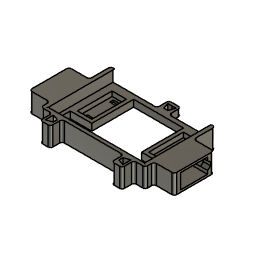
RobotV3 (Autodesk Fusion 360 design; units mm, degrees)
Autodesk Fusion 360 part; units mm, degrees
note: some values were not read from the file. Set by a fixed rule: which sketch regions a step uses.
sketch "Sketch1" plane through (0, 0, 0) normal (0, 0, 1) x (1, 0, 0)
  line L0 (0, 0) -> (83.7, 0)
  line L1 (83.7, 0) -> (83.7, 54.9)
  line L2 (83.7, 54.9) -> (0, 54.9)
  line L3 (0, 54.9) -> (0, 0)
  line L4 (0, 27.45) -> (0, 33.45)
  line L5 (0, 33.45) -> (-1.8, 33.45)
  line L6 (-1.8, 33.45) -> (-25.3, 33.45)
  line L7 (-25.3, 33.45) -> (-25.3, 10.78)
  line L8 (-25.3, 10.78) -> (0, 10.78)
  line L9 (-1.8, 33.45) -> (-1.8, 10.78)
  line L10 (-25.3, 33.45) -> (-25.3, 38.65)
  line L11 (-25.3, 38.65) -> (0, 38.65)
  line L12 (-1.8, 33.45) -> (-1.8, 38.65)
  line L13 (-25.3, 38.65) -> (0, 38.65)
  line L14 (0, 38.65) -> (0, 40.45)
  line L15 (0, 40.45) -> (-25.3, 40.45)
  line L16 (-25.3, 40.45) -> (-25.3, 38.65)
  line L17 (-21.6, 33.45) -> (-18.8, 33.45)
  line L18 (-18.8, 33.45) -> (-18.8, 38.65)
  line L19 (-18.8, 38.65) -> (-21.6, 38.65)
  line L20 (-21.6, 38.65) -> (-21.6, 33.45)
  line L21 (0, 10.78) -> (0, 5.58)
  line L22 (0, 10.78) -> (-18.8, 10.78)
  line L23 (-18.8, 10.78) -> (-18.8, 5.58)
  line L24 (-18.8, 5.58) -> (0, 5.58)
  line L25 (0, 5.58) -> (0, 10.78)
  line L26 (-1.8, 10.78) -> (-1.8, 5.58)
  line L27 (-18.8, 10.78) -> (-21.6, 10.78)
  line L28 (-21.6, 10.78) -> (-21.6, 5.58)
  line L29 (-21.6, 5.58) -> (-18.8, 5.58)
  line L30 (-18.8, 5.58) -> (-18.8, 10.78)
  line L31 (-21.6, 10.78) -> (-25.3, 10.78)
  line L32 (-25.3, 10.78) -> (-25.3, 5.58)
  line L33 (-25.3, 5.58) -> (-21.6, 5.58)
  line L34 (-21.6, 5.58) -> (-21.6, 10.78)
  line L35 (0, 5.58) -> (-25.3, 5.58)
  line L36 (-25.3, 5.58) -> (-25.3, 3.78)
  line L37 (-25.3, 3.78) -> (0, 3.78)
  line L38 (0, 3.78) -> (0, 5.58)
  line L39 (-1.8, 38.65) -> (0, 38.65)
  line L40 (0, 38.65) -> (0, 54.9)
  line L41 (0, 54.9) -> (-1.8, 54.9)
  line L42 (-1.8, 54.9) -> (-1.8, 38.65)
  line L43 (-1.8, 54.9) -> (83.7, 54.9)
  line L44 (83.7, 54.9) -> (83.7, 56.7)
  line L45 (83.7, 56.7) -> (-1.8, 56.7)
  line L46 (-1.8, 56.7) -> (-1.8, 54.9)
  line L47 (0, 0) -> (83.7, 0)
  line L48 (83.7, 0) -> (83.7, -1.8)
  line L49 (83.7, -1.8) -> (0, -1.8)
  line L50 (0, -1.8) -> (0, 0)
  line L51 (83.7, 56.7) -> (85.5, 56.7)
  line L52 (85.5, 56.7) -> (85.5, -1.8)
  line L53 (85.5, -1.8) -> (83.7, -1.8)
  line L54 (83.7, -1.8) -> (83.7, 56.7)
  line L55 (41.85, -1.8) -> (41.85, 56.7)
  line L56 (102.5, 5.58) -> (83.7, 5.58)
  line L57 (109, 5.58) -> (105.3, 5.58)
  line L58 (85.5, 54.9) -> (85.5, 38.65)
  line L59 (85.5, 33.45) -> (85.5, 10.78)
  line L60 (105.3, 33.45) -> (102.5, 33.45)
  line L61 (109, 33.45) -> (109, 10.78)
  line L62 (105.3, 10.78) -> (105.3, 5.58)
  line L63 (105.3, 10.78) -> (109, 10.78)
  line L64 (109, 40.45) -> (109, 38.65)
  line L65 (85.5, 38.65) -> (83.7, 38.65)
  line L66 (109, 33.45) -> (109, 38.65)
  line L67 (105.3, 5.58) -> (102.5, 5.58)
  line L68 (85.5, 10.78) -> (85.5, 5.58)
  line L69 (109, 10.78) -> (109, 5.58)
  line L70 (102.5, 33.45) -> (102.5, 38.65)
  line L71 (102.5, 10.78) -> (102.5, 5.58)
  line L72 (105.3, 5.58) -> (105.3, 10.78)
  line L73 (105.3, 38.65) -> (105.3, 33.45)
  line L74 (102.5, 38.65) -> (105.3, 38.65)
  line L75 (102.5, 5.58) -> (102.5, 10.78)
  line L76 (109, 5.58) -> (109, 3.78)
  line L77 (85.5, 33.45) -> (109, 33.45)
  line L78 (85.5, 33.45) -> (85.5, 38.65)
  line L79 (102.5, 10.78) -> (105.3, 10.78)
  line L80 (85.5, 56.7) -> (85.5, 54.9)
  line L81 (83.7, 38.65) -> (83.7, 54.9)
  line L82 (109, 10.78) -> (83.7, 10.78)
  line L83 (83.7, 3.78) -> (83.7, 5.58)
  line L84 (83.7, 33.45) -> (85.5, 33.45)
  line L85 (109, 3.78) -> (83.7, 3.78)
  line L86 (83.7, 27.45) -> (83.7, 33.45)
  line L87 (83.7, 38.65) -> (83.7, 40.45)
  line L88 (83.7, -1.8) -> (83.7, 0)
  line L89 (83.7, 54.9) -> (83.7, 0)
  line L90 (109, 38.65) -> (83.7, 38.65)
  line L91 (83.7, 10.78) -> (102.5, 10.78)
  line L92 (83.7, 40.45) -> (109, 40.45)
  line L93 (109, 38.65) -> (83.7, 38.65)
  line L94 (83.7, 54.9) -> (85.5, 54.9)
  line L95 (83.7, 5.58) -> (109, 5.58)
  line L96 (83.7, 10.78) -> (83.7, 5.58)
  line L97 (83.7, 5.58) -> (83.7, 10.78)
  line L98 (-1.8, 5.58) -> (0, 5.58)
  line L99 (0, 5.58) -> (0, -1.8)
  line L100 (0, -1.8) -> (-1.8, -1.8)
  line L101 (-1.8, -1.8) -> (-1.8, 5.58)
  line L102 (-18.8, 38.65) -> (-18.8, 40.45)
  line L103 (-18.8, 5.58) -> (-18.8, 3.78)
  line L104 (102.5, 38.65) -> (102.5, 40.45)
  line L105 (102.5, 5.58) -> (102.5, 3.78)
  line L106 (-18.8, 33.45) -> (-18.8, 10.78)
  line L107 (102.5, 33.45) -> (102.5, 10.78)
  point P0 (83.7, 0)
  dimension "d1" = 83.7
  dimension "d2" = 54.9
  dimension "d3" = 6
  dimension "d5" = 1.8
  dimension "d6" = 23.5
  dimension "d7" = 22.67
  dimension "d8" = 5.2
  dimension "d9" = 1.8
  dimension "d10" = 2.8
  dimension "d11" = 17
  dimension "d12" = 5.2
  dimension "d14" = 5.2
  dimension "d15" = 17
  dimension "d16" = 2.8
  dimension "d17" = 5.2
  dimension "d18" = 1.8
  dimension "d19" = 1.8
  dimension "d20" = 1.8
  dimension "d21" = 1.8
  constraint horizontal L0
  constraint vertical L1
  constraint horizontal L2
  constraint vertical L3
  constraint coincident L0.start L3.end
  constraint midpoint L3 L4.start
  constraint parallel L3 L4
  constraint perpendicular L4 L5
  constraint parallel L5 L6
  constraint perpendicular L6 L7
  constraint coincident L3 L8.end
  constraint perpendicular L3 L8
  constraint coincident L8 L9.end
  constraint perpendicular L8 L9
  constraint perpendicular L6 L10
  constraint coincident L3 L11.end
  constraint perpendicular L3 L11
  constraint coincident L11 L12.end
  constraint perpendicular L11 L12
  constraint horizontal L13
  constraint vertical L14
  constraint horizontal L15
  constraint vertical L16
  constraint coincident L3 L14.end
  constraint horizontal L17
  constraint vertical L18
  constraint horizontal L19
  constraint vertical L20
  constraint coincident L6 L17.start
  constraint perpendicular L8 L21
  constraint horizontal L22
  constraint vertical L23
  constraint horizontal L24
  constraint vertical L25
  constraint coincident L24 L26.end
  constraint perpendicular L24 L26
  constraint horizontal L27
  constraint vertical L28
  constraint horizontal L29
  constraint vertical L30
  constraint horizontal L31
  constraint vertical L32
  constraint horizontal L33
  constraint vertical L34
  constraint horizontal L35
  constraint vertical L36
  constraint horizontal L37
  constraint vertical L38
  constraint horizontal L39
  constraint vertical L40
  constraint horizontal L41
  constraint vertical L42
  constraint horizontal L43
  constraint vertical L44
  constraint horizontal L45
  constraint vertical L46
  constraint horizontal L47
  constraint vertical L48
  constraint horizontal L49
  constraint vertical L50
  constraint horizontal L51
  constraint vertical L52
  constraint horizontal L53
  constraint vertical L54
  constraint midpoint L49 L55.start
  constraint coincident L45 L55.end
  constraint perpendicular L45 L55
  constraint symmetric L0.start L55 L0.end
  constraint symmetric L0.start L55 P0
  constraint symmetric L2.end L55 L1.end
  constraint symmetric L4.start L55 L86.start
  constraint symmetric L4.end L55 L84.start
  constraint symmetric L5.end L55 L59.start
  constraint symmetric L6.end L55 L61.start
  constraint symmetric L7.end L55 L61.end
  constraint symmetric L8.end L55 L82.end
  constraint symmetric L9.end L55 L59.end
  constraint symmetric L10.end L55 L64.end
  constraint symmetric L11.end L55 L65.end
  constraint symmetric L12.end L55 L58.end
  constraint symmetric L14.end L55 L87.end
  constraint symmetric L15.end L55 L64.start
  constraint symmetric L17.start L55 L60.start
  constraint symmetric L17.end L55 L60.end
  constraint symmetric L18.end L55 L70.end
  constraint symmetric L19.end L55 L73.start
  constraint symmetric L21.end L55 L56.end
  constraint symmetric L22.end L55 L71.start
  constraint symmetric L23.end L55 L56.start
  constraint symmetric L26.end L55 L68.end
  constraint symmetric L27.end L55 L62.start
  constraint symmetric L28.end L55 L57.end
  constraint symmetric L32.end L55 L57.start
  constraint symmetric L36.end L55 L76.end
  constraint symmetric L37.end L55 L83.start
  constraint symmetric L41.end L55 L58.start
  constraint symmetric L45.end L55 L51.end
  constraint symmetric L49.end L55 L48.end
  constraint horizontal L98
  constraint vertical L99
  constraint horizontal L100
  constraint vertical L101
  constraint coincident L15 L102.end
  constraint perpendicular L15 L102
  constraint coincident L37 L103.end
  constraint perpendicular L37 L103
  constraint coincident L92 L104.end
  constraint perpendicular L92 L104
  constraint coincident L85 L105.end
  constraint perpendicular L85 L105
  measures "d1" distance of L0.start P0
  measures "d2" distance of L0.start L2.end
  measures "d3" distance of L4.start L4.end
  measures "d5" distance of L4.end L5.end
  measures "d6" distance of L5.end L6.end
  measures "d7" distance of L6.end L7.end
  measures "d8" distance of L6.end L10.end
  measures "d9" distance of L10.end L15.end
  measures "d10" distance of L17.start L17.end
  measures "d11" distance of L12 L18
  measures "d12" distance of L8.end L21.end
  measures "d14" distance of L8.end L21.end
  measures "d15" distance of L23 L26
  measures "d16" distance of L22.end L27.end
  measures "d17" distance of L22.end L23.end
  measures "d18" distance of L21.end L37.end
  measures "d19" distance of L41.end L45.end
  measures "d20" distance of L0.start L49.end
  measures "d21" distance of L44.end L51.end
extrude "Extrude1" add sketch "Sketch1" along normal blind 1 contours L0 L2 L3 L4 L14 L21 L25 L38 L40 L43 L47 L55 L99 | L3 L37 L50 L99 L100 L101 | L0 L47 L49 L50 L55 L99 | L0 L1 L2 L43 L47 L54 L55 L81 L83 L86 L87 L89 L96 L97 | L0 L47 L48 L49 L54 L55 L88 | L3 L24 L35 L37 L38 L98 L99 L101 | L1 L48 L52 L53 L54 L85 L88 L89 | L2 L43 L44 L45 L54 L55 | L2 L41 L43 L45 L46 L55 | L3 L8 L21 L22 L24 L25 L26 L35 L98 | L1 L52 L54 L56 L83 L85 L89 L95 | L1 L52 L54 L58 L81 L89 L92 L94 | L44 L51 L52 L54 L80 L94 | L3 L15 L40 L41 L42 L43 | L3 L4 L5 L8 L9 L22 | L8 L22 L23 L24 L26 L30 L35 | L1 L52 L54 L56 L68 L82 L89 L91 L95 L96 L97 | L1 L52 L54 L58 L65 L81 L87 L89 L90 L92 L93 | L3 L11 L13 L14 L15 L39 L40 L42 | L6 L8 L9 L22 L106 | L1 L52 L54 L59 L82 L84 L86 L89 L91 | L52 L56 L68 L71 L75 L82 L91 L95 | L1 L52 L54 L65 L78 L84 L89 L90 L93 | L3 L5 L11 L12 L13 L39 | L6 L11 L12 L13 L18 | L52 L59 L77 L82 L91 L107 | L52 L70 L77 L78 L90 L93
extrude "Extrude2" add sketch "Sketch1" along normal blind 13.3 contours L3 L37 L50 L99 L100 L101 | L0 L47 L49 L50 L55 L99 | L0 L47 L48 L49 L54 L55 L88 | L3 L24 L35 L37 L38 L98 L99 L101 | L1 L48 L52 L53 L54 L85 L88 L89 | L2 L43 L44 L45 L54 L55 | L2 L41 L43 L45 L46 L55 | L3 L8 L21 L22 L24 L25 L26 L35 L98 | L1 L52 L54 L56 L83 L85 L89 L95 | L1 L52 L54 L58 L81 L89 L92 L94 | L44 L51 L52 L54 L80 L94 | L3 L15 L40 L41 L42 L43 | L3 L4 L5 L8 L9 L22 | L8 L22 L23 L24 L26 L30 L35 | L1 L52 L54 L56 L68 L82 L89 L91 L95 L96 L97 | L1 L52 L54 L58 L65 L81 L87 L89 L90 L92 L93 | L3 L11 L13 L14 L15 L39 L40 L42 | L1 L52 L54 L59 L82 L84 L86 L89 L91 | L52 L56 L68 L71 L75 L82 L91 L95 | L1 L52 L54 L65 L78 L84 L89 L90 L93 | L3 L5 L11 L12 L13 L39 | L6 L11 L12 L13 L18 | L52 L70 L77 L78 L90 L93
sketch "Sketch3" plane through (0, 0, 13.3) normal (0, 0, 1) x (-1, 0, 0)
  line L0 (0, 0) -> (0, -54.9)
  line L1 (0, -54.9) -> (-83.7, -54.9)
  line L2 (-83.7, -54.9) -> (-83.7, 0)
  line L3 (-83.7, 0) -> (0, 0)
  line L4 (-85.5, -5.58) -> (-102.5, -5.58)
  line L5 (-102.5, -5.58) -> (-102.5, -10.78)
  line L6 (-102.5, -10.78) -> (-85.5, -10.78)
  line L7 (-85.5, -10.78) -> (-85.5, -33.45)
  line L8 (-85.5, -33.45) -> (-102.5, -33.45)
  line L9 (-102.5, -33.45) -> (-102.5, -38.65)
  line L10 (-102.5, -38.65) -> (-85.5, -38.65)
  line L11 (-85.5, -38.65) -> (-85.5, -56.7)
  line L12 (-85.5, -56.7) -> (1.8, -56.7)
  line L13 (1.8, -56.7) -> (1.8, -38.65)
  line L14 (1.8, -38.65) -> (18.8, -38.65)
  line L15 (18.8, -38.65) -> (18.8, -33.45)
  line L16 (18.8, -33.45) -> (1.8, -33.45)
  line L17 (1.8, -33.45) -> (1.8, -10.78)
  line L18 (1.8, -10.78) -> (18.8, -10.78)
  line L19 (18.8, -10.78) -> (18.8, -5.58)
  line L20 (18.8, -5.58) -> (1.8, -5.58)
  line L21 (1.8, -5.58) -> (1.8, 1.8)
  line L22 (1.8, 1.8) -> (-85.5, 1.8)
  line L23 (-85.5, 1.8) -> (-85.5, -5.58)
  line L24 (18.8, -38.65) -> (0, -38.65)
  line L25 (0, -38.65) -> (0, -5.5037)
  line L26 (0, -5.5037) -> (18.8, -5.5037)
  line L27 (18.8, -5.5037) -> (18.8, -38.65)
  line L28 (-83.7, -38.65) -> (-102.5, -38.65)
  line L29 (-102.5, -38.65) -> (-102.5, -5.58)
  line L30 (-102.5, -5.58) -> (-83.7, -5.58)
  line L31 (-83.7, -5.58) -> (-83.7, -38.65)
  constraint horizontal L24
  constraint vertical L25
  constraint horizontal L26
  constraint vertical L27
  constraint coincident L0 L25.end
  constraint coincident L14.end L15.start
  constraint horizontal L28
  constraint vertical L29
  constraint horizontal L30
  constraint vertical L31
  constraint coincident L4.end L5.start
  constraint coincident L2 L28.start
extrude "Extrude5" add sketch "Sketch3" along normal blind 1 contours L0 L2 L3 L21 L22 L23 L26 L30 | L0 L14 L15 L16 L17 L18 L19 L20 L21 L24 L25 L26 L27 | L0 L1 L2 L11 L12 L13 L24 L28 | L2 L4 L5 L6 L7 L8 L9 L10 L28 L29 L30 L31 | L16 L17 L18 L27 | L6 L7 L8 L29
extrude "Extrude6" add 1 faces at (27.9, 36.6, 1) along direction (0, 0, 1) blind 3.8
sketch "Sketch4" plane through (0, 0, 4.8) normal (0, 0, 1) x (-1, 0, 0)
  line L0 (0, 0) -> (-83.7, 0)
  line L1 (-83.7, 0) -> (-83.7, -54.9)
  line L2 (-83.7, -54.9) -> (0, -54.9)
  line L3 (0, -54.9) -> (0, 0)
  line L4 (-6, -50) -> (-77.7, -50)
  line L5 (-77.7, -50) -> (-77.7, -21)
  line L6 (-77.7, -21) -> (-6, -21)
  line L7 (-6, -21) -> (-6, -50)
  line L8 (-83.7, 0) -> (-83.7, -54.9)
  line L9 (0, -38.65) -> (0, -54.9)
  line L10 (-9, -48) -> (-15, -48)
  line L11 (-15, -48) -> (-15, -45)
  line L12 (-15, -45) -> (-9, -45)
  line L13 (-9, -45) -> (-9, -48)
  line L14 (-21, -48) -> (-21, -45)
  line L15 (-74.7, -48) -> (-68.7, -48)
  line L16 (-68.7, -48) -> (-68.7, -45)
  line L17 (-68.7, -45) -> (-74.7, -45)
  line L18 (-74.7, -45) -> (-74.7, -48)
  line L19 (-9, -26.35) -> (-15, -26.35)
  line L20 (-15, -26.35) -> (-15, -23.35)
  line L21 (-15, -23.35) -> (-9, -23.35)
  line L22 (-9, -23.35) -> (-9, -26.35)
  line L23 (-68.7, -26.35) -> (-74.7, -26.35)
  line L24 (-74.7, -26.35) -> (-74.7, -23.35)
  line L25 (-74.7, -23.35) -> (-68.7, -23.35)
  line L26 (-68.7, -23.35) -> (-68.7, -26.35)
  line L27 (-18, -50) -> (-18, -21)
  line L28 (-65.7, -50) -> (-65.7, -21)
  dimension "d34" = 6
  dimension "d35" = 6
  dimension "d36" = 6
  dimension "d37" = 3
  dimension "d38" = 3
  dimension "d39" = 3
  dimension "d40" = 18.65
  dimension "d41" = 18.65
  dimension "d42" = 6.9
  dimension "d43" = 6.9
  dimension "d44" = 3
  dimension "d45" = 29
  dimension "d48" = 3
  dimension "d49" = 3
  dimension "d50" = 3
  dimension "d51" = 3
  dimension "d52" = 6
  dimension "d53" = 3
  dimension "d123" = 3
  dimension "d124" = 6
  constraint horizontal L4
  constraint vertical L5
  constraint horizontal L6
  constraint vertical L7
  constraint horizontal L10
  constraint vertical L11
  constraint horizontal L12
  constraint vertical L13
  constraint vertical L14
  constraint horizontal L15
  constraint vertical L16
  constraint horizontal L17
  constraint vertical L18
  constraint horizontal L19
  constraint vertical L20
  constraint horizontal L21
  constraint vertical L22
  constraint horizontal L23
  constraint vertical L24
  constraint horizontal L25
  constraint vertical L26
  constraint coincident L4 L27.start
  constraint coincident L6 L27.end
  constraint perpendicular L6 L27
  constraint coincident L4 L28.start
  constraint coincident L6 L28.end
  constraint perpendicular L6 L28
  measures "d34" distance of L5 L8
  measures "d35" distance of L7 L9
  measures "d36" distance of L10.start L10.end
  measures "d37" distance of L10.start L12.end
  measures "d38" distance of L19.start L21.end
  measures "d39" distance of L23.start L25.end
  measures "d40" distance of L12 L19
  measures "d41" distance of L17 L23
  measures "d42" distance of L2 L15
  measures "d43" distance of L2 L10
  measures "d44" distance of L15 L17
  measures "d45" distance of L4 L6
  measures "d48" distance of L11 L27
  measures "d49" distance of L7 L13
  measures "d50" distance of L5 L18
  measures "d51" distance of L5 L24
  measures "d52" distance of L24 L26
  measures "d53" distance of L26 L28
  measures "d123" distance of L7 L22
  measures "d124" distance of L16 L18
extrude "Extrude7" cut sketch "Sketch4" against normal blind 18 contours L10 L11 L12 L13 | L15 L16 L17 L18 | L19 L20 L21 L22 | L23 L24 L25 L26
extrude "Extrude8" cut sketch "Sketch4" against normal blind 4 contours L4 L6 L7 L27 | L4 L5 L6 L28
sketch "Sketch7" plane through (0, 0, 0) normal (0, 0, 1) x (1, 0, 0)
  line L0 (41.8154, -1.8) -> (9.3154, -1.8)
  line L1 (9.3154, -1.8) -> (9.3154, -10)
  line L2 (9.3154, -10) -> (41.8154, -10)
  line L3 (41.8154, -10) -> (41.8154, -1.8)
  line L4 (41.8154, -1.8) -> (74.3154, -1.8)
  line L5 (74.3154, -1.8) -> (74.3154, -10)
  line L6 (74.3154, -10) -> (41.8154, -10)
  line L7 (41.8154, -10) -> (41.8154, -1.8)
  line L8 (9.3154, -1.8) -> (7.5154, -1.8)
  line L9 (7.5154, -1.8) -> (7.5154, -10)
  line L10 (7.5154, -10) -> (9.3154, -10)
  line L11 (9.3154, -10) -> (9.3154, -1.8)
  line L12 (74.3154, -1.8) -> (76.1154, -1.8)
  line L13 (76.1154, -1.8) -> (76.1154, -10)
  line L14 (76.1154, -10) -> (74.3154, -10)
  line L15 (74.3154, -10) -> (74.3154, -1.8)
  line L16 (7.5154, -10) -> (76.1154, -10)
  line L17 (76.1154, -10) -> (76.1154, -11.8)
  line L18 (76.1154, -11.8) -> (7.5154, -11.8)
  line L19 (7.5154, -11.8) -> (7.5154, -10)
  line L20 (9.3154, -5.9) -> (9.3154, -9.3)
  line L21 (9.3154, -5.9) -> (9.3154, -2.5)
  line L22 (9.3154, -9.3) -> (14.3153, -7.6)
  line L23 (9.3154, -9.3) -> (4.0344, -9.3) construction
  line L24 (9.3154, -2.5) -> (14.3153, -4.2)
  line L25 (9.3154, -2.5) -> (4.0344, -2.5) construction
  line L26 (14.3153, -7.6) -> (14.3153, -4.2)
  line L27 (74.3154, -9.3) -> (69.3155, -7.6)
  line L28 (69.3155, -7.6) -> (69.3155, -4.2)
  line L29 (74.3154, -2.5) -> (69.3155, -4.2)
  line L30 (74.3154, -1.8) -> (74.3154, -10)
  line L31 (94, 57) -> (94, 56)
  line L32 (98, 0) -> (98, 55)
  line L33 (98, 27.5) -> (-22.8665, 27.5)
  line L34 (7.5154, 65) -> (76.1154, 65)
  line L35 (76.1154, 56.8) -> (76.1154, 65)
  line L36 (9.3154, 56.8) -> (7.5154, 56.8)
  line L37 (9.3154, 64.3) -> (14.3153, 62.6)
  line L38 (9.3154, 60.9) -> (9.3154, 64.3)
  line L39 (74.3154, 56.8) -> (76.1154, 56.8)
  line L40 (74.3154, 56.8) -> (74.3154, 65)
  line L41 (7.5154, 66.8) -> (7.5154, 65)
  line L42 (41.8154, 56.8) -> (9.3154, 56.8)
  line L43 (9.3154, 56.8) -> (9.3154, 65)
  line L44 (14.3153, 62.6) -> (14.3153, 59.2)
  line L45 (74.3154, 65) -> (41.8154, 65)
  line L46 (76.1154, 66.8) -> (7.5154, 66.8)
  line L47 (41.8154, 56.8) -> (74.3154, 56.8)
  line L48 (9.3154, 65) -> (9.3154, 56.8)
  line L49 (41.8154, 65) -> (41.8154, 56.8)
  line L50 (7.5154, 56.8) -> (7.5154, 65)
  line L51 (74.3154, 64.3) -> (69.3155, 62.6)
  line L52 (9.3154, 57.5) -> (14.3153, 59.2)
  line L53 (9.3154, 57.5) -> (4.0344, 57.5) construction
  line L54 (74.3154, 57.5) -> (69.3155, 59.2)
  line L55 (9.3154, 64.3) -> (4.0344, 64.3) construction
  line L56 (9.3154, 65) -> (41.8154, 65)
  line L57 (74.3154, 65) -> (74.3154, 56.8)
  line L58 (69.3155, 62.6) -> (69.3155, 59.2)
  line L59 (9.3154, 60.9) -> (9.3154, 57.5)
  line L60 (41.8154, 65) -> (41.8154, 56.8)
  line L61 (76.1154, 65) -> (74.3154, 65)
  line L62 (74.3154, 56.8) -> (74.3154, 65)
  line L63 (7.5154, 65) -> (9.3154, 65)
  line L64 (76.1154, 65) -> (76.1154, 66.8)
  dimension "d56" = 32.5
  dimension "d57" = 8.2
  dimension "d58" = 8.2
  dimension "d59" = 1.8
  dimension "d60" = 1.8
  dimension "d61" = 1.8
  dimension "d62" = 32.5
  dimension "d63" = 3.4
  dimension "d64" = 3.4
  dimension "d65" = 161.222
  dimension "d66" = 5.281
  dimension "d67" = 161.222
  dimension "d68" = 5.281
  dimension "d69" = 68.6
  constraint horizontal L0
  constraint vertical L1
  constraint horizontal L2
  constraint vertical L3
  constraint horizontal L4
  constraint vertical L5
  constraint horizontal L6
  constraint vertical L7
  constraint horizontal L8
  constraint vertical L9
  constraint horizontal L10
  constraint vertical L11
  constraint horizontal L12
  constraint vertical L13
  constraint horizontal L14
  constraint vertical L15
  constraint horizontal L16
  constraint vertical L17
  constraint horizontal L18
  constraint vertical L19
  constraint midpoint L1 L20.start
  constraint perpendicular L18 L20
  constraint perpendicular L2 L21
  constraint horizontal L23
  constraint horizontal L25
  constraint symmetric L0.end L3 L4.end
  constraint symmetric L1.end L3 L5.end
  constraint symmetric L3 L20.end L27.start
  constraint symmetric L3 L21.end L29.start
  constraint symmetric L3 L22.end L27.end
  constraint symmetric L3 L24.end L28.end
  constraint vertical L31
  constraint vertical L32
  constraint midpoint L32 L33.start
  constraint perpendicular L32 L33
  constraint symmetric L0.start L33 L42.start
  constraint symmetric L0.end L33 L36.start
  constraint symmetric L1.end L33 L43.end
  constraint symmetric L2.end L33 L45.end
  constraint symmetric L4.end L33 L39.start
  constraint symmetric L5.end L33 L40.end
  constraint symmetric L8.end L33 L36.end
  constraint symmetric L9.end L33 L34.start
  constraint symmetric L12.end L33 L35.start
  constraint symmetric L13.end L33 L34.end
  constraint symmetric L17.end L33 L46.start
  constraint symmetric L18.end L33 L41.start
  constraint symmetric L20.start L33 L38.start
  constraint symmetric L20.end L33 L37.start
  constraint symmetric L21.end L33 L52.start
  constraint symmetric L22.end L33 L37.end
  constraint symmetric L23.end L33 L55.end
  constraint symmetric L24.end L33 L44.end
  constraint symmetric L25.end L33 L53.end
  constraint symmetric L27.start L33 L51.start
  constraint symmetric L27.end L33 L51.end
  constraint symmetric L28.end L33 L54.end
  constraint symmetric L29.start L33 L54.start
  measures "d56" distance of L0.start L0.end
  measures "d57" distance of L0.start L2.end
  measures "d58" distance of L0.start L2.end
  measures "d59" distance of L0.end L8.end
  measures "d60" distance of L4.end L12.end
  measures "d61" distance of L9.end L18.end
  measures "d62" distance of L3 L15
  measures "d63" distance of L20.start L20.end
  measures "d64" distance of L20.start L21.end
  measures "d65" angle of L22 L23
  measures "d66" distance of L20.end L22.end
  measures "d67" angle of L24 L25
  measures "d68" distance of L21.end L24.end
  measures "d69" distance of L17 L19
extrude "Extrude9" add sketch "Sketch7" along normal blind 14.3 contours L0 L1 L2 L3 L7 L11 L16 L22 L24 L26 | L3 L4 L5 L6 L7 L15 L16 L27 L28 L29 L30 | L1 L8 L9 L10 L11 L16 L20 L21 | L2 L6 L10 L14 L16 L17 L18 L19 | L5 L12 L13 L14 L15 L16 L30
sketch "Sketch8" plane through (0, 0, 14.3) normal (0, 0, 1) x (-1, 0, 0)
  line L0 (-9.3154, 9.3) -> (-9.3154, 2.5)
  line L1 (-9.3154, 2.5) -> (-14.3153, 4.2)
  line L2 (-14.3153, 4.2) -> (-14.3153, 7.6)
  line L3 (-14.3153, 7.6) -> (-9.3154, 9.3)
  line L4 (-74.3154, 2.5) -> (-74.3154, 9.3)
  line L5 (-74.3154, 9.3) -> (-69.3155, 7.6)
  line L6 (-69.3155, 7.6) -> (-69.3155, 4.2)
  line L7 (-69.3155, 4.2) -> (-74.3154, 2.5)
  line L8 (-83.7, -54.9) -> (-83.7, 0)
  line L9 (-83.7, 0) -> (0, 0)
  line L10 (0, 0) -> (0, -54.9)
  line L11 (0, -54.9) -> (-83.7, -54.9)
  line L12 (-85.5, -38.65) -> (-85.5, -56.7)
  line L13 (-85.5, -56.7) -> (1.8, -56.7)
  line L14 (1.8, -56.7) -> (1.8, -38.65)
  line L15 (1.8, -38.65) -> (18.8, -38.65)
  line L16 (18.8, -38.65) -> (18.8, -5.58)
  line L17 (18.8, -5.58) -> (1.8, -5.58)
  line L18 (1.8, -5.58) -> (1.8, 1.8)
  line L19 (1.8, 1.8) -> (-7.5154, 1.8)
  line L20 (-7.5154, 1.8) -> (-7.5154, 11.8)
  line L21 (-7.5154, 11.8) -> (-76.1154, 11.8)
  line L22 (-76.1154, 11.8) -> (-76.1154, 1.8)
  line L23 (-76.1154, 1.8) -> (-85.5, 1.8)
  line L24 (-85.5, 1.8) -> (-85.5, -5.58)
  line L25 (-85.5, -5.58) -> (-102.5, -5.58)
  line L26 (-102.5, -5.58) -> (-102.5, -38.65)
  line L27 (-102.5, -38.65) -> (-85.5, -38.65)
  line L28 (-85.5, 1.8) -> (1.8, 1.8)
  line L29 (1.8, 1.8) -> (1.8, -56.7)
  line L30 (1.8, -56.7) -> (-85.5, -56.7)
  line L31 (-85.5, -56.7) -> (-85.5, 1.8)
  line L32 (-1.7, -53.2) -> (-82, -53.2)
  line L33 (-82, -53.2) -> (-82, -1.7)
  line L34 (-82, -1.7) -> (-1.7, -1.7)
  line L35 (-1.7, -1.7) -> (-1.7, -53.2)
  dimension "d72" = 3.5
  constraint horizontal L28
  constraint vertical L29
  constraint horizontal L30
  constraint vertical L31
  constraint coincident L13.end L14.start
  constraint coincident L23.end L24.start
sketch "Sketch10" plane through (0, 56.7, 0) normal (0, 1, 0) x (-1, 0, 0)
  line L0 (-85.5, 0) -> (1.8, 0)
  line L1 (1.8, 0) -> (1.8, 14.3)
  line L2 (-85.5, 14.3) -> (-85.5, 0)
  line L3 (1.8, 14.3) -> (-85.5, 14.3)
extrude "Extrude12" add 1 faces at (-13.1333, 16.6033, 14.3) along direction (0, 0, 1) blind 0.9
sketch "Sketch11" plane through (0, 56.7, 0) normal (0, 1, 0) x (-1, 0, 0)
  line L0 (-83.7, 14.2) -> (0, 14.2)
  line L1 (0, 14.2) -> (0, 4.8)
  line L2 (0, 4.8) -> (-83.7, 4.8)
  line L3 (-83.7, 4.8) -> (-83.7, 14.2)
  line L4 (-85.5, 14.3) -> (-85.5, 0)
  line L5 (1.8, 0) -> (1.8, 14.3)
  line L6 (-83.7, 0) -> (1.8, 0)
  line L7 (-83.7, 14.2) -> (-83.7, 15.2)
  line L8 (-83.7, 15.2) -> (-82.2, 15.2)
  line L9 (-82.2, 15.2) -> (-83.7, 14.2)
  line L10 (0, 14.2) -> (0, 15.2)
  line L11 (0, 15.2) -> (-1.5, 15.2)
  line L12 (-1.5, 15.2) -> (0, 14.2)
  line L13 (-82.2, 15.2) -> (-1.5, 15.2)
  dimension "d85" = 1.8
  dimension "d86" = 1.8
  dimension "d87" = 4.8
  dimension "d89" = 1
  dimension "d90" = 1.5
  dimension "d91" = 1.5
  constraint horizontal L0
  constraint vertical L1
  constraint horizontal L2
  constraint vertical L3
  constraint perpendicular L0 L7
  constraint perpendicular L7 L8
  constraint perpendicular L0 L10
  constraint perpendicular L1 L11
  constraint perpendicular L10 L13
  measures "d85" distance of L3 L4
  measures "d86" distance of L1 L5
  measures "d87" distance of L2 L6
  measures "d89" distance of L0.start L7.end
  measures "d90" distance of L7.end L8.end
  measures "d91" distance of L10.end L11.end
extrude "Extrude13" cut sketch "Sketch11" against normal blind 6 contours L0 L1 L2 L3
extrude "Extrude14" add sketch "Sketch11" against normal blind 58 contours L7 L8 L9 | L10 L11 L12
sketch "Sketch13" plane through (85.5, 0, 0) normal (1, 0, 0) x (0, 1, 0)
  line L0 (-1.8, 0) -> (5.58, 0)
  line L1 (5.58, 0) -> (5.58, 15.2)
  line L2 (5.58, 15.2) -> (-1.8, 15.2)
  line L3 (-1.8, 15.2) -> (-1.8, 0)
  line L4 (0, 15.2) -> (1, 15.2)
  line L5 (0, 15.2) -> (0, 14.2)
  line L6 (0, 14.2) -> (1, 15.2)
  dimension "d96" = 1
  constraint coincident L2 L4.start
  constraint perpendicular L4 L5
  measures "d96" distance of L4.start L4.end
extrude "Extrude15" add sketch "Sketch13" against normal blind 86 contours L2 L4 L5 L6
extrude "Extrude16" cut sketch "Sketch11" against normal blind 4 contours L0 L9 L12 L13
sketch "Sketch14" plane through (0, 0, 4.8) normal (0, 0, 1) x (-1, 0, 0)
  line L0 (-80.7, -3) -> (-3, -3)
  line L1 (-3, -3) -> (-3, -18)
  line L2 (-3, -18) -> (-80.7, -18)
  line L3 (-80.7, -18) -> (-80.7, -3)
  line L4 (-62.7, -18) -> (-21, -18)
  line L5 (-21, -18) -> (-21, -53)
  line L6 (-21, -53) -> (-62.7, -53)
  line L7 (-62.7, -53) -> (-62.7, -18)
  line L8 (-83.7, 0) -> (-83.7, -54.9)
  line L9 (0, -54.9) -> (0, 0)
  line L10 (0, 0) -> (-83.7, 0)
  line L11 (-18, -50) -> (-18, -21)
  line L12 (-65.7, -50) -> (-65.7, -21)
  dimension "d101" = 3
  dimension "d102" = 3
  dimension "d103" = 3
  dimension "d121" = 3
  dimension "d122" = 3
  constraint horizontal L0
  constraint vertical L1
  constraint horizontal L2
  constraint vertical L3
  constraint horizontal L4
  constraint vertical L5
  constraint horizontal L6
  constraint vertical L7
  constraint coincident L2 L4.start
  measures "d101" distance of L3 L8
  measures "d102" distance of L1 L9
  measures "d103" distance of L0 L10
  measures "d121" distance of L5 L11
  measures "d122" distance of L7 L12
extrude "Extrude17" cut sketch "Sketch14" against normal blind 6
sketch "Sketch15" plane through (0, 0, 15.2) normal (0, 0, 1) x (-1, 0, 0)
  line L0 (-1.5, -1) -> (-1.5, -56.7)
  line L1 (-1.5, -56.7) -> (1.8, -56.7)
  line L2 (1.8, -56.7) -> (1.8, -38.65)
  line L3 (1.8, -38.65) -> (18.8, -38.65)
  line L4 (18.8, -38.65) -> (18.8, -5.58)
  line L5 (18.8, -5.58) -> (1.8, -5.58)
  line L6 (1.8, -5.58) -> (1.8, 1.8)
  line L7 (1.8, 1.8) -> (-7.5154, 1.8)
  line L8 (-7.5154, 1.8) -> (-7.5154, 11.8)
  line L9 (-7.5154, 11.8) -> (-76.1154, 11.8)
  line L10 (-76.1154, 11.8) -> (-76.1154, 1.8)
  line L11 (-76.1154, 1.8) -> (-85.5, 1.8)
  line L12 (-85.5, 1.8) -> (-85.5, -5.58)
  line L13 (-85.5, -5.58) -> (-102.5, -5.58)
  line L14 (-102.5, -5.58) -> (-102.5, -38.65)
  line L15 (-102.5, -38.65) -> (-85.5, -38.65)
  line L16 (-85.5, -38.65) -> (-85.5, -56.7)
  line L17 (-85.5, -56.7) -> (-82.2, -56.7)
  line L18 (-82.2, -56.7) -> (-82.2, -1)
  line L19 (-82.2, -1) -> (-1.5, -1)
  line L20 (-74.3154, 2.5) -> (-74.3154, 9.3)
  line L21 (-74.3154, 9.3) -> (-69.3155, 7.6)
  line L22 (-69.3155, 7.6) -> (-69.3155, 4.2)
  line L23 (-69.3155, 4.2) -> (-74.3154, 2.5)
  line L24 (-9.3154, 9.3) -> (-9.3154, 2.5)
  line L25 (-9.3154, 2.5) -> (-14.3153, 4.2)
  line L26 (-14.3153, 4.2) -> (-14.3153, 7.6)
  line L27 (-14.3153, 7.6) -> (-9.3154, 9.3)
  line L28 (-67.5155, 11.8) -> (-16.1153, 11.8)
  line L29 (-16.1153, 11.8) -> (-16.1153, 2)
  line L30 (-16.1153, 2) -> (-67.5155, 2)
  line L31 (-67.5155, 2) -> (-67.5155, 11.8)
  dimension "d106" = 1.8
  dimension "d107" = 1.8
  dimension "d108" = 3
  constraint horizontal L28
  constraint vertical L29
  constraint horizontal L30
  constraint vertical L31
  constraint coincident L9 L28.start
  measures "d106" distance of L22 L31
  measures "d107" distance of L26 L29
  measures "d108" distance of L19 L30
extrude "Extrude18" cut sketch "Sketch15" against normal blind 20 contours L9 L28 L29 L30 L31
sketch "Sketch16" plane through (0, 38.65, 0) normal (0, 1, 0) x (-1, 0, 0)
  line L0 (-102.5, 0) -> (-85.5, 0)
  line L1 (-85.5, 0) -> (-85.5, 15.2)
  line L2 (-85.5, 15.2) -> (-102.5, 15.2)
  line L3 (-102.5, 15.2) -> (-102.5, 0)
  line L4 (-87.5, 10.65) -> (-96.5, 10.65)
  line L5 (-96.5, 10.65) -> (-96.5, 3.55)
  line L6 (-96.5, 3.55) -> (-87.5, 3.55)
  line L7 (-87.5, 3.55) -> (-87.5, 10.65)
  line L8 (-85.5, 14.3) -> (-85.5, 0)
  line L9 (-83.7, 0) -> (-109, 0)
  line L10 (3.8, 10.65) -> (12.8, 10.65)
  line L11 (12.8, 10.65) -> (12.8, 3.55)
  line L12 (12.8, 3.55) -> (3.8, 3.55)
  line L13 (3.8, 3.55) -> (3.8, 10.65)
  line L14 (1.8, 0) -> (1.8, 14.3)
  line L15 (0, 0) -> (25.3, 0)
  dimension "d111" = 9
  dimension "d112" = 2
  dimension "d113" = 4.55
  dimension "d114" = 3.55
  dimension "d115" = 9
  dimension "d116" = 7.1
  dimension "d117" = 2
  dimension "d118" = 3.55
  constraint horizontal L4
  constraint vertical L5
  constraint horizontal L6
  constraint vertical L7
  constraint horizontal L10
  constraint vertical L11
  constraint horizontal L12
  constraint vertical L13
  measures "d111" distance of L4.start L4.end
  measures "d112" distance of L7 L8
  measures "d113" distance of L2 L4
  measures "d114" distance of L6 L9
  measures "d115" distance of L10.start L10.end
  measures "d116" distance of L10.start L12.end
  measures "d117" distance of L13 L14
  measures "d118" distance of L12 L15
extrude "Extrude19" cut sketch "Sketch16" against normal blind 10 contours L4 L5 L6 L7 | L10 L11 L12 L13
sketch "Sketch17" plane through (102.5, 0, 0) normal (1, 0, 0) x (0, 1, 0)
  line L0 (5.58, 15.2) -> (5.58, 0)
  line L1 (5.58, 0) -> (38.65, 0)
  line L2 (38.65, 0) -> (38.65, 15.2)
  line L3 (38.65, 15.2) -> (5.58, 15.2)
  line L4 (10.78, 13.3) -> (33.45, 13.3)
  line L5 (33.45, 13.3) -> (33.45, 1)
  line L6 (33.45, 1) -> (10.78, 1)
  line L7 (10.78, 1) -> (10.78, 13.3)
extrude "Extrude20" add 1 faces at (-11.5333, 20.7433, 0) along direction (0, 0, -1) blind 0.9
sketch "Sketch18" plane through (-18.8, 0, 0) normal (-1, 0, 0) x (0, -1, 0)
  line L0 (-10.78, 13.3) -> (-10.78, 1)
  line L1 (-10.78, 1) -> (-33.45, 1)
  line L2 (-33.45, 1) -> (-33.45, 13.3)
  line L3 (-33.45, 13.3) -> (-10.78, 13.3)
  line L4 (-5.58, -0.9) -> (-5.58, 15.2)
  line L5 (-5.58, 15.2) -> (-38.65, 15.2)
  line L6 (-38.65, 15.2) -> (-38.65, -0.9)
  line L7 (-38.65, -0.9) -> (-5.58, -0.9)
  line L8 (-33.45, 10.65) -> (-36, 10.65)
  line L9 (-36, 10.65) -> (-36, 3.65)
  line L10 (-36, 3.65) -> (-33.45, 3.65)
  line L11 (-33.45, 3.65) -> (-33.45, 10.65)
  line L12 (-33.45, 10.65) -> (-36.0051, 8.506)
  line L13 (-33.45, 10.65) -> (-30.1146, 10.65) construction
  line L14 (-33.45, 3.65) -> (-36, 5.7897)
  line L15 (-33.45, 3.65) -> (-30.1212, 3.65) construction
  dimension "d127" = 2.55
  dimension "d128" = 4.55
  dimension "d129" = 4.55
  dimension "d139" = 140
  dimension "d140" = 140
  constraint horizontal L8
  constraint vertical L9
  constraint horizontal L10
  constraint vertical L11
  constraint coincident L2 L8.start
  constraint horizontal L13
  constraint horizontal L15
  constraint coincident L9 L14.end
  measures "d127" distance of L8.start L8.end
  measures "d128" distance of L5 L8
  measures "d129" distance of L7 L10
  measures "d139" angle of L12 L13
  measures "d140" angle of L14 L15
extrude "Extrude23" cut sketch "Sketch18" against normal blind 8 contours L2 L9 L11 L12 L14
sketch "Sketch20" plane through (102.5, 0, 0) normal (1, 0, 0) x (0, 1, 0)
  line L0 (33.45, 10.65) -> (33.45, 3.65)
  line L1 (33.45, 3.65) -> (36, 5.79)
  line L2 (36, 5.79) -> (36, 8.51)
  line L3 (36, 8.51) -> (33.45, 10.65)
  constraint vertical L0
  constraint parallel L0 L2
extrude "Extrude24" cut sketch "Sketch20" against normal blind 8
sketch "Sketch21" plane through (102.5, 0, 0) normal (1, 0, 0) x (0, 1, 0)
  line L0 (10.78, 13.3) -> (33.45, 13.3)
  line L1 (33.45, 13.3) -> (33.45, 1)
  line L2 (33.45, 1) -> (10.78, 1)
  line L3 (10.78, 1) -> (10.78, 13.3)
  line L4 (10.78, 13.3) -> (33.45, 13.3)
  line L5 (33.45, 13.3) -> (33.45, 13.4)
  line L6 (33.45, 13.4) -> (10.78, 13.4)
  line L7 (10.78, 13.4) -> (10.78, 13.3)
  line L8 (33.45, 1) -> (10.78, 1)
  line L9 (10.78, 1) -> (10.78, 0.9)
  line L10 (10.78, 0.9) -> (33.45, 0.9)
  line L11 (33.45, 0.9) -> (33.45, 1)
  dimension "d145" = 0.1
  dimension "d146" = 0.1
  constraint horizontal L0
  constraint vertical L1
  constraint horizontal L2
  constraint vertical L3
  constraint horizontal L4
  constraint vertical L5
  constraint horizontal L6
  constraint vertical L7
  constraint horizontal L8
  constraint vertical L9
  constraint horizontal L10
  constraint vertical L11
  measures "d145" distance of L0.start L6.end
  measures "d146" distance of L1.end L10.end
extrude "Extrude25" cut sketch "Sketch21" against normal blind 17 contours L0 L4 L5 L6 L7 | L2 L8 L9 L10 L11
sketch "Sketch22" plane through (-18.8, 0, 0) normal (-1, 0, 0) x (0, -1, 0)
  line L0 (-33.45, 13.3) -> (-10.78, 13.3)
  line L1 (-10.78, 13.3) -> (-10.78, 13.4)
  line L2 (-10.78, 13.4) -> (-33.45, 13.4)
  line L3 (-33.45, 13.4) -> (-33.45, 13.3)
  line L4 (-33.45, 1) -> (-10.78, 1)
  line L5 (-10.78, 1) -> (-10.78, 0.9)
  line L6 (-10.78, 0.9) -> (-33.45, 0.9)
  line L7 (-33.45, 0.9) -> (-33.45, 1)
  dimension "d149" = 0.1
  dimension "d150" = 0.1
  constraint horizontal L0
  constraint vertical L1
  constraint horizontal L2
  constraint vertical L3
  constraint horizontal L4
  constraint vertical L5
  constraint horizontal L6
  constraint vertical L7
  measures "d149" distance of L0.start L2.end
  measures "d150" distance of L4.start L6.end
extrude "Extrude26" cut sketch "Sketch22" against normal blind 17
sketch "Sketch25" plane through (0, 0, -0.9) normal (0, 0, -1) x (1, 0, 0)
  line L0 (67.5155, 11.8) -> (67.5155, 2)
  line L1 (67.5155, 2) -> (16.1153, 2)
  line L2 (16.1153, 2) -> (16.1153, 11.8)
  line L3 (16.1153, 11.8) -> (7.5154, 11.8)
  line L4 (7.5154, 11.8) -> (7.5154, 1.8)
  line L5 (7.5154, 1.8) -> (-1.8, 1.8)
  line L6 (-1.8, 1.8) -> (-1.8, -5.58)
  line L7 (-1.8, -5.58) -> (-18.8, -5.58)
  line L8 (-18.8, -5.58) -> (-18.8, -38.65)
  line L9 (-18.8, -38.65) -> (-1.8, -38.65)
  line L10 (-1.8, -38.65) -> (-1.8, -56.7)
  line L11 (-1.8, -56.7) -> (85.5, -56.7)
  line L12 (85.5, -56.7) -> (85.5, -38.65)
  line L13 (85.5, -38.65) -> (102.5, -38.65)
  line L14 (102.5, -38.65) -> (102.5, -5.58)
  line L15 (102.5, -5.58) -> (85.5, -5.58)
  line L16 (85.5, -5.58) -> (85.5, 1.8)
  line L17 (85.5, 1.8) -> (76.1154, 1.8)
  line L18 (76.1154, 1.8) -> (76.1154, 11.8)
  line L19 (76.1154, 11.8) -> (67.5155, 11.8)
  line L20 (15, -23.35) -> (15, -26.35)
  line L21 (15, -26.35) -> (9, -26.35)
  line L22 (9, -26.35) -> (9, -23.35)
  line L23 (9, -23.35) -> (15, -23.35)
  line L24 (15, -45) -> (15, -48)
  line L25 (15, -48) -> (9, -48)
  line L26 (9, -48) -> (9, -45)
  line L27 (9, -45) -> (15, -45)
  line L28 (74.7, -23.35) -> (74.7, -26.35)
  line L29 (74.7, -26.35) -> (68.7, -26.35)
  line L30 (68.7, -26.35) -> (68.7, -23.35)
  line L31 (68.7, -23.35) -> (74.7, -23.35)
  line L32 (74.7, -48) -> (68.7, -48)
  line L33 (68.7, -48) -> (68.7, -45)
  line L34 (68.7, -45) -> (74.7, -45)
  line L35 (74.7, -45) -> (74.7, -48)
  line L36 (74.3154, 9.3) -> (74.3154, 2.5)
  line L37 (74.3154, 2.5) -> (69.3155, 4.2)
  line L38 (69.3155, 4.2) -> (69.3155, 7.6)
  line L39 (69.3155, 7.6) -> (74.3154, 9.3)
  line L40 (9.3154, 2.5) -> (9.3154, 9.3)
  line L41 (9.3154, 9.3) -> (14.3153, 7.6)
  line L42 (14.3153, 7.6) -> (14.3153, 4.2)
  line L43 (14.3153, 4.2) -> (9.3154, 2.5)
  line L44 (21, -53) -> (21, -18)
  line L45 (21, -18) -> (3, -18)
  line L46 (3, -18) -> (3, -3)
  line L47 (3, -3) -> (80.7, -3)
  line L48 (80.7, -3) -> (80.7, -18)
  line L49 (80.7, -18) -> (62.7, -18)
  line L50 (62.7, -18) -> (62.7, -53)
  line L51 (62.7, -53) -> (21, -53)
  line L52 (41.85, -56.7) -> (46.85, -56.7)
  line L53 (46.85, -56.7) -> (46.85, -66.7)
  line L54 (46.85, -66.7) -> (41.85, -66.7)
  line L55 (41.85, -66.7) -> (41.85, -56.7)
  line L56 (41.85, -66.7) -> (36.85, -66.7)
  line L57 (36.85, -66.7) -> (36.85, -56.7)
  line L58 (36.85, -56.7) -> (41.85, -56.7)
  line L59 (41.85, -56.7) -> (41.85, -66.7)
  line L60 (41.85, -64.2) -> (38.45, -64.2)
  line L61 (41.85, -64.2) -> (45.25, -64.2)
  line L62 (45.25, -64.2) -> (43.5481, -59.2007)
  line L63 (45.25, -64.2) -> (39.969, -64.2) construction
  line L64 (38.45, -64.2) -> (40.1519, -59.2007)
  line L65 (38.45, -64.2) -> (43.731, -64.2) construction
  line L66 (43.5481, -59.2007) -> (40.1519, -59.2007)
  dimension "d157" = 5
  dimension "d158" = 10
  dimension "d159" = 5
  dimension "d160" = 10
  dimension "d162" = 3.4
  dimension "d163" = 3.4
  dimension "d164" = 71.2
  dimension "d165" = 5.281
  dimension "d166" = 71.2
  dimension "d167" = 5.281
  dimension "d168" = 2.5
  constraint horizontal L52
  constraint vertical L53
  constraint horizontal L54
  constraint vertical L55
  constraint midpoint L11 L52.start
  constraint horizontal L56
  constraint vertical L57
  constraint horizontal L58
  constraint vertical L59
  constraint coincident L59 L60.start
  constraint perpendicular L59 L60
  constraint perpendicular L55 L61
  constraint horizontal L63
  constraint horizontal L65
  measures "d157" distance of L52.start L52.end
  measures "d158" distance of L52.start L54.end
  measures "d159" distance of L54.end L56.end
  measures "d160" distance of L54.end L52.start
  measures "d162" distance of L60.start L60.end
  measures "d163" distance of L60.start L61.end
  measures "d164" angle of L62 L63
  measures "d165" distance of L61.end L62.end
  measures "d166" angle of L64 L65
  measures "d167" distance of L60.end L64.end
  measures "d168" distance of L56 L65
extrude "Extrude27" add sketch "Sketch25" against normal blind 5.7 contours L11 L52 L53 L54 L55 L59 L61 L62 L66 | L11 L55 L56 L57 L58 L59 L60 L64 L66
fillet "Fillet4" radius 2 20 edges at (-1.8, 56.7, 7.15) (-1.8, 38.65, 7.15) (-18.8, 38.65, 7.15) (-18.8, 5.58, 7.15) (-1.8, 5.58, 7.15) (-1.8, -1.8, 7.15) (7.5154, -1.8, 7.15) (7.5154, -11.8, 7.15) (16.1153, -11.8, 7.15) (16.1153, -2, 7.15) (67.5155, -2, 7.15) (67.5155, -11.8, 7.15) (76.1154, -11.8, 7.15) (76.1154, -1.8, 7.15) (85.5, -1.8, 7.15) (85.5, 5.58, 7.15) (102.5, 5.58, 7.15) (102.5, 38.65, 7.15) (85.5, 38.65, 7.15) (85.5, 56.7, 7.15)
fillet "Fillet5" radius 2 4 edges at (46.85, 56.7, 1.95) (46.85, 66.7, 1.95) (36.85, 66.7, 1.95) (36.85, 56.7, 1.95)
sketch "Sketch26" plane through (0, 56.7, 0) normal (0, 1, 0) x (-1, 0, 0)
  line L0 (-48.85, -0.9) -> (-48.85, 4.8)
  line L1 (-48.85, 4.8) -> (-83.5, 4.8)
  line L2 (-83.5, 4.8) -> (-83.5, -0.9)
  line L3 (-83.5, -0.9) -> (-48.85, -0.9)
equation "d1 = 83.5 mm + 0.2 mm"
equation "d2 = 54.7 mm + 0.2 mm"
equation "d6 = 23.3 mm + 0.2 mm"
equation "d7 = 22.47 mm + 0.2 mm"
equation "d24 = 12.3 mm + 1 mm"
equation "d32 = 13.3 mm - 9.5 mm"
equation "d56 = ( 65 / 2 ) * 1 mm"
equation "d62 = ( 65 / 2 ) * 1 mm"
equation "d63 = ( 6.8 / 2 ) * 1 mm"
equation "d64 = ( 6.8 / 2 ) * 1 mm"
equation "d65 = 90 deg + 71.222 deg"
equation "d67 = 71.222 deg + 90 deg"
equation "d69 = ( ( 32.5 + 1.8 ) * 2 ) * 1 mm"
equation "d113 = ( ( 16.1 - 7 ) / 2 ) * 1 mm"
equation "d164 = 161.2 deg - 90 deg"
